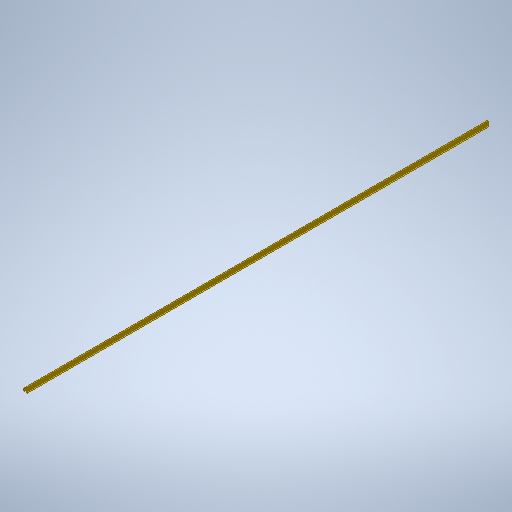
# Autodesk Inventor part: Perfil 20×20 R90 2 rasgos
Saved by Autodesk Inventor 2025.2 (Build 292293000, 293)
## iProperties
Created: 2025-03-28
Part Number: Perfil 20×20 R90 2 rasgos
Material: Ouro
Document SubType Name: Modeling
Designer: lucas
Density: 19.3 g/cm^3
Appearance: Metal quente 2400F
Author: lucas
Autodesk Inventor part; units mm, degrees
ref_plane "YZ Plane" through (0, 0, 0) normal (1, 0, 0) x (0, 1, 0)
ref_plane "XZ Plane" through (0, 0, 0) normal (0, 1, 0) x (-1, 0, 0)
ref_plane "XY Plane" through (0, 0, 0) normal (0, 0, 1) x (1, 0, 0)
sketch "Esboço2" plane through (0, 0, 0) normal (0, 0, 1) x (1, 0, 0)
  circle A0 centre (0, 0) radius 2.5
  line L0 (10, 10) -> (10, -10) construction
  line L1 (10, 3.1) -> (10, -3.1) construction
  line L2 (4, 3.1) -> (4, -3.1) construction
  line L3 (0, 0) -> (2.5, 0) construction
  line L4 (10, 10) -> (10, 3.1) construction
  line L5 (10, 3.1) -> (8, 3.1) construction
  line L6 (8, 3.1) -> (8, 6.8) construction
  line L7 (8, 6.8) -> (4, 3.1) construction
  line L8 (10, -3.1) -> (10, -10) construction
  line L9 (8, -3.1) -> (10, -3.1) construction
  line L10 (8, -3.1) -> (8, -6.8) construction
  line L11 (8, -6.8) -> (4, -3.1) construction
  line L12 (10, 3.1) -> (9.5, 3.1) construction
  line L13 (9.5, 3.1) -> (9.5, 3.6)
  line L14 (9.5, 3.6) -> (10, 3.6)
  line L15 (10, 3.6) -> (10, 3.1) construction
  line L16 (10, 10) -> (10, 3.6) construction
  line L17 (9.5, 3.1) -> (8, 3.1)
  line L18 (10, -3.1) -> (9.5, -3.1) construction
  line L19 (9.5, -3.1) -> (9.5, -3.6)
  line L20 (9.5, -3.6) -> (10, -3.6)
  line L21 (10, -3.6) -> (10, -3.1) construction
  line L22 (10, -3.6) -> (10, -10) construction
  line L23 (8, -3.1) -> (9.5, -3.1)
  line L24 (0, 0) -> (0, -2.5) construction
  line L25 (0, 2.5) -> (0, 0) construction
  arc A1 (10, 9.5) -> (9.5, 10) centre (9.5, 9.5) ccw
  line L26 (10, 9.5) -> (10, 3.6)
  line L27 (-10, 10) -> (10, 10) construction
  line L28 (-10, 10) -> (-10, -10) construction
  line L29 (0, 0) -> (-10, 10) construction
  line L30 (-2.5, 0) -> (0, 0) construction
  arc A2 (8, 5.6564) -> (7.1605, 6.0234) centre (7.5, 5.6564) ccw
  line L31 (8, 5.6564) -> (8, 3.1)
  arc A3 (7.1605, -6.0234) -> (8, -5.6564) centre (7.5, -5.6564) ccw
  arc A4 (4.1605, 3.2484) -> (4, 2.8814) centre (4.5, 2.8814) ccw
  arc A5 (4, -2.8814) -> (4.1605, -3.2484) centre (4.5, -2.8814) ccw
  line L32 (4, 2.8814) -> (4, -2.8814)
  line L33 (4.1605, -3.2484) -> (7.1605, -6.0234)
  line L34 (4.1605, 3.2484) -> (7.1605, 6.0234)
  line L35 (8, -3.1) -> (8, -5.6564)
  arc A6 (9.5, -10) -> (10, -9.5) centre (9.5, -9.5) ccw
  line L36 (10, -3.6) -> (10, -9.5)
  arc A7 (9.5, 10) -> (-10, -9.5) centre (9.5, -9.5) ccw
  arc A8 (-10, -9.5) -> (-9.5, -10) centre (-9.5, -9.5) ccw
  line L37 (-3.1, 4.3108) -> (3.1, 4.3108) construction
  line L38 (3.1, 4.3108) -> (8, 8.8433) construction
  arc A9 (6.8948, 7.821) -> (6.4827, 8.6828) centre (6.5553, 8.1881) ccw
  arc A10 (2.9042, 4.3108) -> (3.2437, 4.4438) centre (2.9042, 4.8108) ccw
  arc A11 (8, 8.8433) -> (-3.1, 4.3108) centre (9.2294, -10.0255) ccw construction
  arc A12 (-1.9647, 5.2138) -> (-1.6687, 4.3108) centre (-1.6687, 4.8108) ccw
  line L39 (-1.6687, 4.3108) -> (2.9042, 4.3108)
  arc A13 (6.4827, 8.6828) -> (-1.9647, 5.2138) centre (9.2294, -10.0255) ccw
  line L40 (3.2437, 4.4438) -> (6.8948, 7.821)
  line L41 (-6.8, -8) -> (-3.1, -8) construction
  line L42 (-10, -10) -> (10, -10) construction
  line L43 (-3.1, -10) -> (3.1, -10) construction
  line L44 (-10, -10) -> (-3.1, -10) construction
  line L45 (-9.5, -10) -> (-3.1, -10) construction
  line L46 (-3.1, -8) -> (-3.1, -10) construction
  line L47 (3.1, -10) -> (10, -10) construction
  line L48 (3.1, -8) -> (3.1, -10) construction
  line L49 (3.1, -8) -> (7.0883, -8) construction
  line L50 (3.1, -10) -> (9.5, -10) construction
  line L51 (2.764, -4) -> (7.0883, -8) construction
  line L52 (-2.764, -4) -> (2.764, -4) construction
  line L53 (-6.8, -8) -> (-2.764, -4) construction
  arc A14 (-5.9372, -7.1449) -> (-5.5852, -8) centre (-5.5852, -7.5) ccw
  arc A15 (-2.5582, -4) -> (-2.9101, -4.1449) centre (-2.5582, -4.5) ccw
  arc A16 (2.9077, -4.133) -> (2.5682, -4) centre (2.5682, -4.5) ccw
  arc A17 (5.8114, -8) -> (6.151, -7.133) centre (5.8114, -7.5) ccw
  line L54 (-3.1, -10) -> (-3.6, -10) construction
  line L55 (-3.6, -10) -> (-3.6, -9.5)
  line L56 (-3.6, -9.5) -> (-3.1, -9.5)
  line L57 (-3.1, -9.5) -> (-3.1, -10) construction
  line L58 (-9.5, -10) -> (-3.6, -10)
  line L59 (-3.1, -9.5) -> (-3.1, -8)
  line L60 (-2.9101, -4.1449) -> (-5.9372, -7.1449)
  line L61 (-2.5582, -4) -> (2.5682, -4)
  line L62 (6.151, -7.133) -> (2.9077, -4.133)
  line L63 (3.1, -8) -> (5.8114, -8)
  line L64 (-5.5852, -8) -> (-3.1, -8)
  line L65 (3.1, -10) -> (3.6, -10) construction
  line L66 (3.6, -10) -> (3.6, -9.5)
  line L67 (3.6, -9.5) -> (3.1, -9.5)
  line L68 (3.1, -9.5) -> (3.1, -10) construction
  line L69 (3.6, -10) -> (9.5, -10)
  line L70 (3.1, -8) -> (3.1, -9.5)
  line L71 (-8.9309, -8) -> (-4, -3.1131) construction
  line L72 (-4, -3.1131) -> (-4, 2.889) construction
  arc A18 (-4, 2.889) -> (-8.9309, -8) centre (9.8766, -9.9556) ccw construction
  arc A19 (-8.7144, -6.503) -> (-7.8708, -6.9494) centre (-8.2228, -6.5943) ccw
  arc A20 (-4, 1.5422) -> (-4.8905, 1.8545) centre (-4.5, 1.5422) ccw
  arc A21 (-4.148, -3.2598) -> (-4, -2.9047) centre (-4.5, -2.9047) ccw
  arc A22 (-4.8863, 1.8598) -> (-8.7144, -6.503) centre (9.8766, -9.9556) ccw
  line L73 (-4, 1.5422) -> (-4, -2.9047)
  line L74 (-4.148, -3.2598) -> (-7.8708, -6.9494)
  point P0 (10, 0)
  point P1 (10, 0)
  point P2 (4, 0)
  point P3 (0, 4.3108)
  point P4 (0, -10)
  point P5 (0, -10)
  point P6 (10, 6.8)
  point P7 (8, -4.3782)
  point P8 (0, -4)
  point P9 (-4.8905, 1.8545)
  dimension "d6" = 5
  dimension "d7" = 20
  dimension "d8" = 10
  dimension "d9" = 6.2
  dimension "d11" = 6
  dimension "d17" = 2
  dimension "d22" = 0.5
  dimension "d24" = 0.5
  dimension "d65" = 1.5
  dimension "d67" = 1.5
  dimension "d69" = 1.5
  dimension "d70" = 1.5
  dimension "d72" = 1.5
  constraints: 150 end point, 51 point on circle, 37 tangent, 31 point on line, 23 centre point, 22 equal length, 20 horizontal, 19 equal radius, 14 vertical, 11 parallel, 9 midpoint, 7 coincident, 4 collinear, 4 horizontal alignment, 4 perpendicular, 3 vertical alignment
  measures "d6" diameter of A0
  measures "d7" distance of L0.start L0.end
  measures "d8" distance from line of L0 point (0, 0)
  measures "d9" distance of L1.end L1.start
  measures "d11" distance between parallel lines of L0 L2
  measures "d17" distance between parallel lines of L4 L6
  measures "d22" distance of L13.end L14.end
  measures "d24" radius of A1
  measures "d65" distance between parallel lines of L7 L38
  measures "d67" distance between parallel lines of L11 L51
  measures "d69" distance from line of L24.end L52
  measures "d70" distance between parallel lines of L60 L71
  measures "d72" distance from line of L30.start L72
extrude "Extrusão1" add sketch "Esboço2" along normal mid plane 2000
